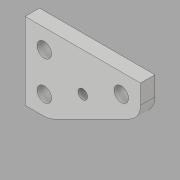
# Autodesk Inventor part: Plate
Saved by Autodesk Inventor 2020 (Build 240168000, 168)
## iProperties
Created: 2017-03-30
Part Number: Plate
Material: Genérico
Document SubType Name: Modeling
Designer: Jorge
Density: 1 g/cm^3
Appearance: Por defecto
Author: Jorge
Autodesk Inventor part; units mm, degrees
ref_plane "YZ Plane" through (0, 0, 0) normal (1, 0, 0) x (0, 1, 0)
ref_plane "XZ Plane" through (0, 0, 0) normal (0, 1, 0) x (-1, 0, 0)
ref_plane "XY Plane" through (0, 0, 0) normal (0, 0, 1) x (1, 0, 0)
sketch "Sketch1" plane through (0, 0, 0) normal (0, 0, 1) x (1, 0, 0)
  line L0 (0, 0) -> (76.2, 0)
  line L1 (0, 0) -> (0, -50.8)
  line L2 (0, -50.8) -> (12.7, -50.8)
  line L3 (18.3796, -49.4592) -> (69.1796, -24.0592)
  arc A0 (12.7, -50.8) -> (18.3796, -49.4592) centre (12.7, -38.1) ccw
  line L4 (76.2, 0) -> (76.2, -12.7)
  arc A1 (69.1796, -24.0592) -> (76.2, -12.7) centre (63.5, -12.7) ccw
  circle A2 centre (12.7, -38.1) radius 4.8006
  circle A3 centre (12.7, -12.7) radius 4.8006
  circle A4 centre (63.5, -12.7) radius 4.8006
  line L5 (12.7, -12.7) -> (63.5, -12.7) construction
  line L6 (12.7, -38.1) -> (12.7, -12.7) construction
  circle A5 centre (38.1, -25.4) radius 3.175
  dimension "d2" = 50.8
  dimension "d3" = 12.7
  dimension "d4" = 12.7
  dimension "d5" = 12.7
  dimension "d7" = 9.6012
  dimension "d8" = 25.4
  dimension "d10" = 50.8
  dimension "d11" = 12.7
  dimension "d12" = 6.35
  dimension "d13" = 12.7
  dimension "d14" = 25.4
  dimension "d15" = 12.7
  dimension "d16" = 76.2
  constraints: 14 end point, 6 centre point, 4 point on circle, 4 tangent, 3 equal radius, 3 horizontal, 2 vertical, 1 perpendicular
  measures "d2" distance of L0.start L1.end
  measures "d3" distance of L1.end L2.end
  measures "d4" radius of A0
  measures "d5" distance of L0.end L4.end
  measures "d7" diameter of A3
  measures "d8" distance of L6.start L5.start
  measures "d10" distance of L5.end L5.start
  measures "d11" distance from line of L1 L5.start
  measures "d12" diameter of A5
  measures "d13" vertical distance of A1.centre A5.centre
  measures "d14" horizontal distance of A5.centre A0.centre
  measures "d15" distance from line of L5.start L0
  measures "d16" distance between parallel lines of L4 L1
extrude "Extrusion1" add sketch "Sketch1" along normal mid plane 9.525
body "Solid1"
